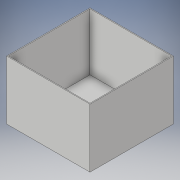
# Autodesk Inventor part: 546-1550Z137-4.8x4.8-Enclosure
Saved by Autodesk Inventor 2018 (Build 220112000, 112)
## iProperties
Created: 2018-04-30
Part Number: 546-1550Z137-4.8x4.8-Enclosure
Material: Generic
Document SubType Name: Modeling
Designer: bbramman
Density: 1 g/cm^3
Appearance: Default
Author: bbramman
Autodesk Inventor part; units mm, degrees
ref_plane "YZ Plane" through (0, 0, 0) normal (1, 0, 0) x (0, 1, 0)
ref_plane "XZ Plane" through (0, 0, 0) normal (0, 1, 0) x (-1, 0, 0)
ref_plane "XY Plane" through (0, 0, 0) normal (0, 0, 1) x (1, 0, 0)
sketch "Sketch1" plane through (0, 0, 0) normal (0, 1, 0) x (-1, 0, 0)
  line L0 (-60.452, -60.452) -> (60.452, -60.452)
  line L1 (60.452, -60.452) -> (60.452, 60.452)
  line L2 (60.452, 60.452) -> (-60.452, 60.452)
  line L3 (-60.452, 60.452) -> (-60.452, -60.452)
  line L4 (-60.452, -60.452) -> (60.452, 60.452) construction
  line L5 (60.452, -60.452) -> (-60.452, 60.452) construction
  point P0 (0, 0)
  dimension "d0" = 120.904
  dimension "d1" = 120.904
  constraints: 12 end point, 2 midpoint, 2 parallel, 1 horizontal, 1 perpendicular
  measures "d0" distance of L2.end L1.end
  measures "d1" distance of L1.end L0.end
extrude "Extrusion1" add sketch "Sketch1" along normal blind 2.54
sketch "Sketch2" plane through (0, 2.54, 0) normal (0, 1, 0) x (1, 0, 0)
  line L0 (60.452, 60.452) -> (-60.452, 60.452) projected
  line L1 (60.452, -60.452) -> (-60.452, -60.452)
  line L2 (-60.452, -60.452) -> (-60.452, 60.452)
  line L3 (-60.452, 60.452) -> (60.452, 60.452)
  line L4 (60.452, 60.452) -> (60.452, -60.452)
  line L5 (60.452, -60.452) -> (-60.452, 60.452) construction
  line L6 (-60.452, -60.452) -> (60.452, 60.452) construction
  line L7 (59.182, -59.182) -> (-59.182, -59.182)
  line L8 (-59.182, -59.182) -> (-59.182, 59.182)
  line L9 (-59.182, 59.182) -> (59.182, 59.182)
  line L10 (59.182, 59.182) -> (59.182, -59.182)
  line L11 (59.182, -59.182) -> (-59.182, 59.182) construction
  line L12 (-59.182, -59.182) -> (59.182, 59.182) construction
  point P0 (0, 0)
  dimension "d4" = 118.364
  dimension "d5" = 118.364
  constraints: 24 end point, 4 midpoint, 4 parallel, 2 horizontal, 2 perpendicular
  measures "d4" distance of L8.end L9.end
  measures "d5" distance of L7.end L8.end
extrude "Extrusion2" add sketch "Sketch2" along normal blind 82.804
sketch "Sketch3" plane through (0, 2.54, 0) normal (0, 1, 0) x (1, 0, 0)
  circle A0 centre (0, -25.4) radius 2.0828
  circle A1 centre (0, 25.4) radius 2.0828
  point P0 (0, 0)
  dimension "d10" = 4.1656
  dimension "d11" = 4.1656
  constraints: 2 centre point
  measures "d10" diameter of A0
  measures "d11" diameter of A1
extrude "Extrusion3" cut sketch "Sketch3" against normal through all
body "Solid1"
